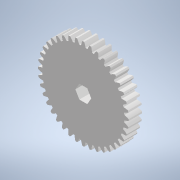
# Autodesk Inventor part: engranaje40
Saved by Autodesk Inventor 2022 (Build 260153000, 153)
## iProperties
Created: 2022-03-10
Part Number: engranaje40
Material: Generic
Document SubType Name: Modeling
Designer: katha
Density: 1 g/cm^3
Appearance: Default
Author: katha
Autodesk Inventor part; units mm, degrees
(part 1 of 4)
ref_plane "YZ Plane" through (0, 0, 0) normal (1, 0, 0) x (0, 1, 0)
ref_plane "XZ Plane" through (0, 0, 0) normal (0, 1, 0) x (-1, 0, 0)
ref_plane "XY Plane" through (0, 0, 0) normal (0, 0, 1) x (1, 0, 0)
sketch "Sketch4" plane through (0, 0, 0) normal (0, 0, 1) x (1, 0, 0)
  circle A0 centre (0, 0) radius 2
  circle A1 centre (0, 0) radius 2
  line L0 (20.6501, 2.8098) -> (20.4934, 2.709)
  line L1 (20.4934, 2.709) -> (20.3445, 2.6176)
  line L2 (20.3445, 2.6176) -> (20.199, 2.5324)
  line L3 (20.199, 2.5324) -> (20.06, 2.4548)
  line L4 (20.06, 2.4548) -> (19.7984, 2.3194)
  line L5 (19.7984, 2.3194) -> (19.561, 2.2088)
  line L6 (19.561, 2.2088) -> (19.3491, 2.1207)
  line L7 (19.3491, 2.1207) -> (19.1647, 2.0529)
  line L8 (19.1647, 2.0529) -> (19.0089, 2.0007)
  line L9 (19.0089, 2.0007) -> (18.9606, 1.9795)
  line L10 (18.9606, 1.9795) -> (18.9216, 1.9573)
  line L11 (18.9216, 1.9573) -> (18.8918, 1.9346)
  line L12 (18.8918, 1.9346) -> (18.8713, 1.9116)
  line L13 (18.8713, 1.9116) -> (18.86, 1.8888)
  line L14 (18.86, 1.8888) -> (18.8579, 1.8665)
  line L15 (18.8579, 1.8665) -> (18.8612, 1.833)
  line L16 (18.8612, 1.833) -> (18.8916, 1.4868)
  line L17 (18.8916, 1.4868) -> (18.9157, 1.1401)
  line L18 (18.9157, 1.1401) -> (18.9177, 1.1065)
  line L19 (18.9177, 1.1065) -> (18.9232, 1.0848)
  line L20 (18.9232, 1.0848) -> (18.938, 1.0641)
  line L21 (18.938, 1.0641) -> (18.9618, 1.0446)
  line L22 (18.9618, 1.0446) -> (18.9948, 1.0268)
  line L23 (18.9948, 1.0268) -> (19.0368, 1.011)
  line L24 (19.0368, 1.011) -> (19.0878, 0.9976)
  line L25 (19.0878, 0.9976) -> (19.2499, 0.9703)
  line L26 (19.2499, 0.9703) -> (19.4426, 0.9323)
  line L27 (19.4426, 0.9323) -> (19.6657, 0.8784)
  line L28 (19.6657, 0.8784) -> (19.9175, 0.8063)
  line L29 (19.9175, 0.8063) -> (20.1971, 0.7134)
  line L30 (20.1971, 0.7134) -> (20.3465, 0.6586)
  line L31 (20.3465, 0.6586) -> (20.5035, 0.5972)
  line L32 (20.5035, 0.5972) -> (20.6649, 0.5302)
  line L33 (20.6649, 0.5302) -> (20.8354, 0.4552)
  line L34 (20.8354, 0.4552) -> (20.9966, 0.3803)
  arc A2 (20.9966, -0.3803) -> (20.9966, 0.3803) centre (0, 0) ccw
  line L35 (20.9966, -0.3803) -> (20.8354, -0.4552)
  line L36 (20.8354, -0.4552) -> (20.6649, -0.5302)
  line L37 (20.6649, -0.5302) -> (20.5035, -0.5972)
  line L38 (20.5035, -0.5972) -> (20.3465, -0.6586)
  line L39 (20.3465, -0.6586) -> (20.1971, -0.7135)
  line L40 (20.1971, -0.7135) -> (19.9175, -0.8063)
  line L41 (19.9175, -0.8063) -> (19.6657, -0.8784)
  line L42 (19.6657, -0.8784) -> (19.4426, -0.9323)
  line L43 (19.4426, -0.9323) -> (19.2499, -0.9703)
  line L44 (19.2499, -0.9703) -> (19.0878, -0.9976)
  line L45 (19.0878, -0.9976) -> (19.0368, -1.011)
  line L46 (19.0368, -1.011) -> (18.9948, -1.0268)
  line L47 (18.9948, -1.0268) -> (18.9618, -1.0446)
  line L48 (18.9618, -1.0446) -> (18.938, -1.0641)
  line L49 (18.938, -1.0641) -> (18.9232, -1.0848)
  line L50 (18.9232, -1.0848) -> (18.9177, -1.1065)
  line L51 (18.9177, -1.1065) -> (18.9157, -1.1401)
  line L52 (18.9157, -1.1401) -> (18.8916, -1.4868)
  line L53 (18.8916, -1.4868) -> (18.8612, -1.833)
  line L54 (18.8612, -1.833) -> (18.8579, -1.8665)
  line L55 (18.8579, -1.8665) -> (18.86, -1.8888)
  line L56 (18.86, -1.8888) -> (18.8713, -1.9116)
  line L57 (18.8713, -1.9116) -> (18.8918, -1.9346)
  line L58 (18.8918, -1.9346) -> (18.9216, -1.9573)
  line L59 (18.9216, -1.9573) -> (18.9606, -1.9795)
  line L60 (18.9606, -1.9795) -> (19.0089, -2.0007)
  line L61 (19.0089, -2.0007) -> (19.1647, -2.053)
  line L62 (19.1647, -2.053) -> (19.3491, -2.1207)
  line L63 (19.3491, -2.1207) -> (19.561, -2.2088)
  line L64 (19.561, -2.2088) -> (19.7984, -2.3194)
  line L65 (19.7984, -2.3194) -> (20.06, -2.4548)
  line L66 (20.06, -2.4548) -> (20.199, -2.5324)
  line L67 (20.199, -2.5324) -> (20.3445, -2.6176)
  line L68 (20.3445, -2.6176) -> (20.4934, -2.709)
  line L69 (20.4934, -2.709) -> (20.6501, -2.8098)
  line L70 (20.6501, -2.8098) -> (20.7975, -2.909)
  arc A3 (20.6786, -3.6602) -> (20.7975, -2.909) centre (0, 0) ccw
  line L71 (20.6786, -3.6602) -> (20.5077, -3.709)
  line L72 (20.5077, -3.709) -> (20.3275, -3.7564)
  line L73 (20.3275, -3.7564) -> (20.1577, -3.7973)
  line L74 (20.1577, -3.7973) -> (19.993, -3.8334)
  line L75 (19.993, -3.8334) -> (19.8368, -3.8642)
  line L76 (19.8368, -3.8642) -> (19.5462, -3.9122)
  line L77 (19.5462, -3.9122) -> (19.2862, -3.944)
  line L78 (19.2862, -3.944) -> (19.0574, -3.9623)
  line L79 (19.0574, -3.9623) -> (18.8611, -3.9697)
  line L80 (18.8611, -3.9697) -> (18.6968, -3.9713)
  line L81 (18.6968, -3.9713) -> (18.6443, -3.9765)
  line L82 (18.6443, -3.9765) -> (18.6003, -3.9856)
  line L83 (18.6003, -3.9856) -> (18.565, -3.998)
  line L84 (18.565, -3.998) -> (18.5383, -4.0135)
  line L85 (18.5383, -4.0135) -> (18.5205, -4.0317)
  line L86 (18.5205, -4.0317) -> (18.5117, -4.0522)
  line L87 (18.5117, -4.0522) -> (18.5045, -4.0852)
  line L88 (18.5045, -4.0852) -> (18.4264, -4.4238)
  line L89 (18.4264, -4.4238) -> (18.3423, -4.761)
  line L90 (18.3423, -4.761) -> (18.3337, -4.7936)
  line L91 (18.3337, -4.7936) -> (18.3323, -4.8159)
  line L92 (18.3323, -4.8159) -> (18.3399, -4.8402)
  line L93 (18.3399, -4.8402) -> (18.3566, -4.8661)
  line L94 (18.3566, -4.8661) -> (18.3824, -4.8932)
  line L95 (18.3824, -4.8932) -> (18.4175, -4.9212)
  line L96 (18.4175, -4.9212) -> (18.4619, -4.9497)
  line L97 (18.4619, -4.9497) -> (18.6076, -5.0257)
  line L98 (18.6076, -5.0257) -> (18.7791, -5.1215)
  line L99 (18.7791, -5.1215) -> (18.9746, -5.2416)
  line L100 (18.9746, -5.2416) -> (19.1918, -5.388)
  line L101 (19.1918, -5.388) -> (19.429, -5.5627)
  line L102 (19.429, -5.5627) -> (19.5542, -5.661)
  line L103 (19.5542, -5.661) -> (19.6846, -5.768)
  line L104 (19.6846, -5.768) -> (19.8173, -5.8815)
  line L105 (19.8173, -5.8815) -> (19.9563, -6.0056)
  line L106 (19.9563, -6.0056) -> (20.0864, -6.1266)
  arc A4 (19.8514, -6.85) -> (20.0864, -6.1266) centre (0, 0) ccw
  line L107 (19.8514, -6.85) -> (19.675, -6.8714)
  line L108 (19.675, -6.8714) -> (19.4896, -6.8901)
  line L109 (19.4896, -6.8901) -> (19.3155, -6.9039)
  line L110 (19.3155, -6.9039) -> (19.1472, -6.9138)
  line L111 (19.1472, -6.9138) -> (18.9881, -6.9198)
  line L112 (18.9881, -6.9198) -> (18.6935, -6.9217)
  line L113 (18.6935, -6.9217) -> (18.4318, -6.9124)
  line L114 (18.4318, -6.9124) -> (18.203, -6.8948)
  line L115 (18.203, -6.8948) -> (18.0079, -6.8714)
  line L116 (18.0079, -6.8714) -> (17.8454, -6.8472)
  line L117 (17.8454, -6.8472) -> (17.7927, -6.8442)
  line L118 (17.7927, -6.8442) -> (17.7479, -6.8462)
  line L119 (17.7479, -6.8462) -> (17.711, -6.853)
  line L120 (17.711, -6.853) -> (17.6823, -6.8641)
  line L121 (17.6823, -6.8641) -> (17.6618, -6.8793)
  line L122 (17.6618, -6.8793) -> (17.6499, -6.8982)
  line L123 (17.6499, -6.8982) -> (17.6376, -6.9296)
  line L124 (17.6376, -6.9296) -> (17.5075, -7.2519)
  line L125 (17.5075, -7.2519) -> (17.3717, -7.5717)
  line L126 (17.3717, -7.5717) -> (17.3581, -7.6026)
  line L127 (17.3581, -7.6026) -> (17.3532, -7.6244)
  line L128 (17.3532, -7.6244) -> (17.3569, -7.6496)
  line L129 (17.3569, -7.6496) -> (17.3694, -7.6778)
  line L130 (17.3694, -7.6778) -> (17.3907, -7.7086)
  line L131 (17.3907, -7.7086) -> (17.4209, -7.7418)
  line L132 (17.4209, -7.7418) -> (17.4603, -7.7769)
  line L133 (17.4603, -7.7769) -> (17.5923, -7.8747)
  line L134 (17.5923, -7.8747) -> (17.7468, -7.9961)
  line L135 (17.7468, -7.9961) -> (17.9211, -8.1454)
  line L136 (17.9211, -8.1454) -> (18.1127, -8.324)
  line L137 (18.1127, -8.324) -> (18.3196, -8.5336)
  line L138 (18.3196, -8.5336) -> (18.4279, -8.6503)
  line L139 (18.4279, -8.6503) -> (18.5399, -8.7763)
  line L140 (18.5399, -8.7763) -> (18.6532, -8.9092)
  line L141 (18.6532, -8.9092) -> (18.7712, -9.0535)
  line L142 (18.7712, -9.0535) -> (18.8807, -9.1934)
  arc A5 (18.5354, -9.8711) -> (18.8807, -9.1934) centre (0, 0) ccw
  line L143 (18.5354, -9.8711) -> (18.3579, -9.8647)
  line L144 (18.3579, -9.8647) -> (18.1718, -9.8541)
  line L145 (18.1718, -9.8541) -> (17.9976, -9.8405)
  line L146 (17.9976, -9.8405) -> (17.8299, -9.8239)
  line L147 (17.8299, -9.8239) -> (17.6718, -9.805)
  line L148 (17.6718, -9.805) -> (17.3806, -9.7608)
  line L149 (17.3806, -9.7608) -> (17.1235, -9.7107)
  line L150 (17.1235, -9.7107) -> (16.9003, -9.6574)
  line L151 (16.9003, -9.6574) -> (16.7112, -9.6038)
  line L152 (16.7112, -9.6038) -> (16.5545, -9.5545)
  line L153 (16.5545, -9.5545) -> (16.503, -9.5433)
  line L154 (16.503, -9.5433) -> (16.4584, -9.5383)
  line L155 (16.4584, -9.5383) -> (16.4209, -9.5392)
  line L156 (16.4209, -9.5392) -> (16.3908, -9.5457)
  line L157 (16.3908, -9.5457) -> (16.3682, -9.5575)
  line L158 (16.3682, -9.5575) -> (16.3535, -9.5743)
  line L159 (16.3535, -9.5743) -> (16.3364, -9.6034)
  line L160 (16.3364, -9.6034) -> (16.1575, -9.9014)
  line L161 (16.1575, -9.9014) -> (15.9733, -10.196)
  line L162 (15.9733, -10.196) -> (15.9551, -10.2244)
  line L163 (15.9551, -10.2244) -> (15.9468, -10.2452)
  line L164 (15.9468, -10.2452) -> (15.9466, -10.2706)
  line L165 (15.9466, -10.2706) -> (15.9544, -10.3004)
  line L166 (15.9544, -10.3004) -> (15.9707, -10.3342)
  line L167 (15.9707, -10.3342) -> (15.9954, -10.3717)
  line L168 (15.9954, -10.3717) -> (16.0287, -10.4125)
  line L169 (16.0287, -10.4125) -> (16.1438, -10.5298)
  line L170 (16.1438, -10.5298) -> (16.2774, -10.6739)
  line L171 (16.2774, -10.6739) -> (16.4262, -10.8486)
  line L172 (16.4262, -10.8486) -> (16.5875, -11.0549)
  line L173 (16.5875, -11.0549) -> (16.7591, -11.2943)
  line L174 (16.7591, -11.2943) -> (16.8478, -11.4266)
  line L175 (16.8478, -11.4266) -> (16.9387, -11.5685)
  line L176 (16.9387, -11.5685) -> (17.0299, -11.7175)
  line L177 (17.0299, -11.7175) -> (17.1238, -11.8785)
  line L178 (17.1238, -11.8785) -> (17.2101, -12.0338)
  arc A6 (16.7631, -12.6491) -> (17.2101, -12.0338) centre (0, 0) ccw
  line L179 (16.7631, -12.6491) -> (16.5887, -12.615)
  line L180 (16.5887, -12.615) -> (16.4066, -12.5755)
  line L181 (16.4066, -12.5755) -> (16.2367, -12.5348)
  line L182 (16.2367, -12.5348) -> (16.0735, -12.4922)
  line L183 (16.0735, -12.4922) -> (15.9204, -12.4487)
  line L184 (15.9204, -12.4487) -> (15.6397, -12.3595)
  line L185 (15.6397, -12.3595) -> (15.3936, -12.2699)
  line L186 (15.3936, -12.2699) -> (15.1815, -12.1823)
  line L187 (15.1815, -12.1823) -> (15.0031, -12.0998)
  line L188 (15.0031, -12.0998) -> (14.856, -12.0266)
  line L189 (14.856, -12.0266) -> (14.8069, -12.0075)
  line L190 (14.8069, -12.0075) -> (14.7636, -11.9956)
  line L191 (14.7636, -11.9956) -> (14.7265, -11.9906)
  line L192 (14.7265, -11.9906) -> (14.6957, -11.9923)
  line L193 (14.6957, -11.9923) -> (14.6716, -12.0004)
  line L194 (14.6716, -12.0004) -> (14.6544, -12.0147)
  line L195 (14.6544, -12.0147) -> (14.633, -12.0408)
  line L196 (14.633, -12.0408) -> (14.4097, -12.307)
  line L197 (14.4097, -12.307) -> (14.1816, -12.5693)
  line L198 (14.1816, -12.5693) -> (14.1592, -12.5944)
  line L199 (14.1592, -12.5944) -> (14.1478, -12.6137)
  line L200 (14.1478, -12.6137) -> (14.1436, -12.6388)
  line L201 (14.1436, -12.6388) -> (14.1467, -12.6694)
  line L202 (14.1467, -12.6694) -> (14.1574, -12.7053)
  line L203 (14.1574, -12.7053) -> (14.1759, -12.7462)
  line L204 (14.1759, -12.7462) -> (14.2025, -12.7918)
  line L205 (14.2025, -12.7918) -> (14.2978, -12.9256)
  line L206 (14.2978, -12.9256) -> (14.4072, -13.0888)
  line L207 (14.4072, -13.0888) -> (14.5269, -13.2846)
  line L208 (14.5269, -13.2846) -> (14.654, -13.5137)
  line L209 (14.654, -13.5137) -> (14.786, -13.777)
  line L210 (14.786, -13.777) -> (14.8529, -13.9214)
  line L211 (14.8529, -13.9214) -> (14.9205, -14.0759)
  line L212 (14.9205, -14.0759) -> (14.9872, -14.2373)
  line L213 (14.9872, -14.2373) -> (15.0547, -14.411)
  line L214 (15.0547, -14.411) -> (15.1157, -14.5779)
  arc A7 (14.5779, -15.1157) -> (15.1157, -14.5779) centre (0, 0) ccw
  line L215 (14.5779, -15.1157) -> (14.411, -15.0547)
  line L216 (14.411, -15.0547) -> (14.2373, -14.9872)
  line L217 (14.2373, -14.9872) -> (14.0759, -14.9205)
  line L218 (14.0759, -14.9205) -> (13.9214, -14.8529)
  line L219 (13.9214, -14.8529) -> (13.777, -14.786)
  line L220 (13.777, -14.786) -> (13.5137, -14.654)
  line L221 (13.5137, -14.654) -> (13.2846, -14.5269)
  line L222 (13.2846, -14.5269) -> (13.0888, -14.4072)
  line L223 (13.0888, -14.4072) -> (12.9256, -14.2978)
  line L224 (12.9256, -14.2978) -> (12.7918, -14.2025)
  line L225 (12.7918, -14.2025) -> (12.7462, -14.176)
  line L226 (12.7462, -14.176) -> (12.7053, -14.1574)
  line L227 (12.7053, -14.1574) -> (12.6694, -14.1467)
  line L228 (12.6694, -14.1467) -> (12.6388, -14.1436)
  line L229 (12.6388, -14.1436) -> (12.6137, -14.1478)
  line L230 (12.6137, -14.1478) -> (12.5944, -14.1592)
  line L231 (12.5944, -14.1592) -> (12.5693, -14.1816)
  line L232 (12.5693, -14.1816) -> (12.307, -14.4097)
  line L233 (12.307, -14.4097) -> (12.0408, -14.633)
  line L234 (12.0408, -14.633) -> (12.0147, -14.6544)
  line L235 (12.0147, -14.6544) -> (12.0004, -14.6716)
  line L236 (12.0004, -14.6716) -> (11.9923, -14.6957)
  line L237 (11.9923, -14.6957) -> (11.9906, -14.7265)
  line L238 (11.9906, -14.7265) -> (11.9956, -14.7636)
  line L239 (11.9956, -14.7636) -> (12.0075, -14.8069)
  line L240 (12.0075, -14.8069) -> (12.0266, -14.856)
  line L241 (12.0266, -14.856) -> (12.0998, -15.0031)
  line L242 (12.0998, -15.0031) -> (12.1823, -15.1815)
  line L243 (12.1823, -15.1815) -> (12.2698, -15.3936)
  line L244 (12.2698, -15.3936) -> (12.3595, -15.6397)
  line L245 (12.3595, -15.6397) -> (12.4487, -15.9204)
  line L246 (12.4487, -15.9204) -> (12.4922, -16.0736)
  line L247 (12.4922, -16.0736) -> (12.5348, -16.2367)
  line L248 (12.5348, -16.2367) -> (12.5755, -16.4066)
  line L249 (12.5755, -16.4066) -> (12.615, -16.5887)
  line L250 (12.615, -16.5887) -> (12.6491, -16.7631)
  arc A8 (12.0338, -17.2101) -> (12.6491, -16.7631) centre (0, 0) ccw
  line L251 (12.0338, -17.2101) -> (11.8785, -17.1238)
  line L252 (11.8785, -17.1238) -> (11.7175, -17.0299)
  line L253 (11.7175, -17.0299) -> (11.5685, -16.9387)
  line L254 (11.5685, -16.9387) -> (11.4265, -16.8478)
  line L255 (11.4265, -16.8478) -> (11.2943, -16.7591)
  line L256 (11.2943, -16.7591) -> (11.0549, -16.5875)
  line L257 (11.0549, -16.5875) -> (10.8486, -16.4262)
  line L258 (10.8486, -16.4262) -> (10.6739, -16.2774)
  line L259 (10.6739, -16.2774) -> (10.5298, -16.1438)
  line L260 (10.5298, -16.1438) -> (10.4125, -16.0287)
  line L261 (10.4125, -16.0287) -> (10.3717, -15.9954)
  line L262 (10.3717, -15.9954) -> (10.3342, -15.9707)
  line L263 (10.3342, -15.9707) -> (10.3004, -15.9544)
  line L264 (10.3004, -15.9544) -> (10.2706, -15.9466)
  line L265 (10.2706, -15.9466) -> (10.2452, -15.9469)
  line L266 (10.2452, -15.9469) -> (10.2244, -15.9551)
  line L267 (10.2244, -15.9551) -> (10.196, -15.9733)
  line L268 (10.196, -15.9733) -> (9.9014, -16.1575)
  line L269 (9.9014, -16.1575) -> (9.6034, -16.3365)
  line L270 (9.6034, -16.3365) -> (9.5743, -16.3535)
  line L271 (9.5743, -16.3535) -> (9.5575, -16.3682)
  line L272 (9.5575, -16.3682) -> (9.5457, -16.3908)
  line L273 (9.5457, -16.3908) -> (9.5392, -16.4209)
  line L274 (9.5392, -16.4209) -> (9.5383, -16.4584)
  line L275 (9.5383, -16.4584) -> (9.5433, -16.503)
  line L276 (9.5433, -16.503) -> (9.5545, -16.5545)
  line L277 (9.5545, -16.5545) -> (9.6038, -16.7112)
  line L278 (9.6038, -16.7112) -> (9.6574, -16.9003)
  line L279 (9.6574, -16.9003) -> (9.7107, -17.1235)
  line L280 (9.7107, -17.1235) -> (9.7608, -17.3806)
  line L281 (9.7608, -17.3806) -> (9.805, -17.6718)
  line L282 (9.805, -17.6718) -> (9.8239, -17.8299)
  line L283 (9.8239, -17.8299) -> (9.8405, -17.9977)
  line L284 (9.8405, -17.9977) -> (9.8541, -18.1718)
  line L285 (9.8541, -18.1718) -> (9.8647, -18.3579)
  line L286 (9.8647, -18.3579) -> (9.8711, -18.5354)
  arc A9 (9.1934, -18.8807) -> (9.8711, -18.5354) centre (0, 0) ccw
  line L287 (9.1934, -18.8807) -> (9.0535, -18.7712)
  line L288 (9.0535, -18.7712) -> (8.9092, -18.6532)
  line L289 (8.9092, -18.6532) -> (8.7763, -18.5399)
  line L290 (8.7763, -18.5399) -> (8.6503, -18.4279)
  line L291 (8.6503, -18.4279) -> (8.5336, -18.3196)
  line L292 (8.5336, -18.3196) -> (8.324, -18.1127)
  line L293 (8.324, -18.1127) -> (8.1454, -17.9211)
  line L294 (8.1454, -17.9211) -> (7.9961, -17.7468)
  line L295 (7.9961, -17.7468) -> (7.8747, -17.5923)
  line L296 (7.8747, -17.5923) -> (7.7769, -17.4603)
  line L297 (7.7769, -17.4603) -> (7.7418, -17.4209)
  line L298 (7.7418, -17.4209) -> (7.7086, -17.3907)
  line L299 (7.7086, -17.3907) -> (7.6778, -17.3694)
  line L300 (7.6778, -17.3694) -> (7.6496, -17.3569)
  line L301 (7.6496, -17.3569) -> (7.6244, -17.3532)
  line L302 (7.6244, -17.3532) -> (7.6026, -17.3581)
  line L303 (7.6026, -17.3581) -> (7.5717, -17.3717)
  line L304 (7.5717, -17.3717) -> (7.2519, -17.5075)
  line L305 (7.2519, -17.5075) -> (6.9296, -17.6376)
  line L306 (6.9296, -17.6376) -> (6.8982, -17.6499)
  line L307 (6.8982, -17.6499) -> (6.8793, -17.6618)
  line L308 (6.8793, -17.6618) -> (6.8641, -17.6823)
  line L309 (6.8641, -17.6823) -> (6.853, -17.711)
  line L310 (6.853, -17.711) -> (6.8462, -17.7479)
  line L311 (6.8462, -17.7479) -> (6.8442, -17.7927)
  line L312 (6.8442, -17.7927) -> (6.8472, -17.8454)
  line L313 (6.8472, -17.8454) -> (6.8714, -18.0079)
  line L314 (6.8714, -18.0079) -> (6.8947, -18.203)
  line L315 (6.8947, -18.203) -> (6.9124, -18.4318)
  line L316 (6.9124, -18.4318) -> (6.9217, -18.6935)
  line L317 (6.9217, -18.6935) -> (6.9198, -18.9881)
  line L318 (6.9198, -18.9881) -> (6.9138, -19.1472)
  line L319 (6.9138, -19.1472) -> (6.9039, -19.3155)
  line L320 (6.9039, -19.3155) -> (6.8901, -19.4896)
  line L321 (6.8901, -19.4896) -> (6.8714, -19.675)
  line L322 (6.8714, -19.675) -> (6.85, -19.8514)
  arc A10 (6.1266, -20.0864) -> (6.85, -19.8514) centre (0, 0) ccw
  line L323 (6.1266, -20.0864) -> (6.0056, -19.9563)
  line L324 (6.0056, -19.9563) -> (5.8815, -19.8173)
  line L325 (5.8815, -19.8173) -> (5.768, -19.6846)
  line L326 (5.768, -19.6846) -> (5.661, -19.5542)
  line L327 (5.661, -19.5542) -> (5.5627, -19.429)
  line L328 (5.5627, -19.429) -> (5.388, -19.1919)
  line L329 (5.388, -19.1919) -> (5.2416, -18.9746)
  line L330 (5.2416, -18.9746) -> (5.1215, -18.7791)
  line L331 (5.1215, -18.7791) -> (5.0257, -18.6076)
  line L332 (5.0257, -18.6076) -> (4.9497, -18.4619)
  line L333 (4.9497, -18.4619) -> (4.9212, -18.4175)
  line L334 (4.9212, -18.4175) -> (4.8932, -18.3825)
  line L335 (4.8932, -18.3825) -> (4.8661, -18.3566)
  line L336 (4.8661, -18.3566) -> (4.8402, -18.3399)
  line L337 (4.8402, -18.3399) -> (4.8159, -18.3323)
  line L338 (4.8159, -18.3323) -> (4.7936, -18.3337)
  line L339 (4.7936, -18.3337) -> (4.761, -18.3423)
  line L340 (4.761, -18.3423) -> (4.4238, -18.4264)
  line L341 (4.4238, -18.4264) -> (4.0852, -18.5045)
  line L342 (4.0852, -18.5045) -> (4.0522, -18.5117)
  line L343 (4.0522, -18.5117) -> (4.0317, -18.5206)
  line L344 (4.0317, -18.5206) -> (4.0135, -18.5383)
  line L345 (4.0135, -18.5383) -> (3.998, -18.565)
  line L346 (3.998, -18.565) -> (3.9856, -18.6004)
  line L347 (3.9856, -18.6004) -> (3.9765, -18.6443)
  line L348 (3.9765, -18.6443) -> (3.9713, -18.6968)
  line L349 (3.9713, -18.6968) -> (3.9697, -18.8611)
  line L350 (3.9697, -18.8611) -> (3.9623, -19.0574)
  line L351 (3.9623, -19.0574) -> (3.944, -19.2862)
  line L352 (3.944, -19.2862) -> (3.9122, -19.5462)
  line L353 (3.9122, -19.5462) -> (3.8642, -19.8368)
  line L354 (3.8642, -19.8368) -> (3.8334, -19.993)
  line L355 (3.8334, -19.993) -> (3.7973, -20.1577)
  line L356 (3.7973, -20.1577) -> (3.7564, -20.3275)
  line L357 (3.7564, -20.3275) -> (3.709, -20.5077)
  line L358 (3.709, -20.5077) -> (3.6602, -20.6786)
  arc A11 (2.909, -20.7975) -> (3.6602, -20.6786) centre (0, 0) ccw
  line L359 (2.909, -20.7975) -> (2.8098, -20.6501)
  line L360 (2.8098, -20.6501) -> (2.709, -20.4934)
  line L361 (2.709, -20.4934) -> (2.6176, -20.3445)
  line L362 (2.6176, -20.3445) -> (2.5324, -20.199)
  line L363 (2.5324, -20.199) -> (2.4548, -20.06)
  line L364 (2.4548, -20.06) -> (2.3194, -19.7984)
  line L365 (2.3194, -19.7984) -> (2.2088, -19.561)
  line L366 (2.2088, -19.561) -> (2.1207, -19.3491)
  line L367 (2.1207, -19.3491) -> (2.0529, -19.1647)
  line L368 (2.0529, -19.1647) -> (2.0007, -19.0089)
  line L369 (2.0007, -19.0089) -> (1.9795, -18.9606)
  line L370 (1.9795, -18.9606) -> (1.9573, -18.9216)
  line L371 (1.9573, -18.9216) -> (1.9346, -18.8918)
  line L372 (1.9346, -18.8918) -> (1.9116, -18.8713)
  line L373 (1.9116, -18.8713) -> (1.8888, -18.86)
  line L374 (1.8888, -18.86) -> (1.8665, -18.8579)
  line L375 (1.8665, -18.8579) -> (1.833, -18.8612)
  line L376 (1.833, -18.8612) -> (1.4868, -18.8916)
  line L377 (1.4868, -18.8916) -> (1.1401, -18.9157)
  line L378 (1.1401, -18.9157) -> (1.1065, -18.9177)
  line L379 (1.1065, -18.9177) -> (1.0848, -18.9232)
  line L380 (1.0848, -18.9232) -> (1.0641, -18.938)
  line L381 (1.0641, -18.938) -> (1.0446, -18.9618)
  line L382 (1.0446, -18.9618) -> (1.0268, -18.9948)
  line L383 (1.0268, -18.9948) -> (1.011, -19.0369)
  line L384 (1.011, -19.0369) -> (0.9976, -19.0878)
  line L385 (0.9976, -19.0878) -> (0.9703, -19.2499)
  line L386 (0.9703, -19.2499) -> (0.9323, -19.4427)
  line L387 (0.9323, -19.4427) -> (0.8784, -19.6657)
  line L388 (0.8784, -19.6657) -> (0.8063, -19.9175)
  line L389 (0.8063, -19.9175) -> (0.7135, -20.1971)
  line L390 (0.7135, -20.1971) -> (0.6586, -20.3465)
  line L391 (0.6586, -20.3465) -> (0.5972, -20.5035)
  line L392 (0.5972, -20.5035) -> (0.5302, -20.6649)
  line L393 (0.5302, -20.6649) -> (0.4552, -20.8354)
  line L394 (0.4552, -20.8354) -> (0.3803, -20.9966)
  arc A12 (-0.3803, -20.9966) -> (0.3803, -20.9966) centre (0, 0) ccw
  line L395 (-0.3803, -20.9966) -> (-0.4552, -20.8354)
  line L396 (-0.4552, -20.8354) -> (-0.5302, -20.6649)
  line L397 (-0.5302, -20.6649) -> (-0.5972, -20.5035)
  line L398 (-0.5972, -20.5035) -> (-0.6586, -20.3465)
  line L399 (-0.6586, -20.3465) -> (-0.7135, -20.1971)
  line L400 (-0.7135, -20.1971) -> (-0.8063, -19.9175)
  line L401 (-0.8063, -19.9175) -> (-0.8784, -19.6657)
  line L402 (-0.8784, -19.6657) -> (-0.9323, -19.4426)
  line L403 (-0.9323, -19.4426) -> (-0.9703, -19.2499)
  line L404 (-0.9703, -19.2499) -> (-0.9976, -19.0878)
  line L405 (-0.9976, -19.0878) -> (-1.011, -19.0369)
  line L406 (-1.011, -19.0369) -> (-1.0268, -18.9948)
  line L407 (-1.0268, -18.9948) -> (-1.0446, -18.9618)
  line L408 (-1.0446, -18.9618) -> (-1.0641, -18.938)
  line L409 (-1.0641, -18.938) -> (-1.0848, -18.9232)
  line L410 (-1.0848, -18.9232) -> (-1.1065, -18.9177)
  line L411 (-1.1065, -18.9177) -> (-1.1401, -18.9157)
  line L412 (-1.1401, -18.9157) -> (-1.4868, -18.8916)
  line L413 (-1.4868, -18.8916) -> (-1.833, -18.8612)
  line L414 (-1.833, -18.8612) -> (-1.8665, -18.8579)
  line L415 (-1.8665, -18.8579) -> (-1.8888, -18.86)
  line L416 (-1.8888, -18.86) -> (-1.9116, -18.8713)
  line L417 (-1.9116, -18.8713) -> (-1.9346, -18.8918)
  line L418 (-1.9346, -18.8918) -> (-1.9573, -18.9216)
  line L419 (-1.9573, -18.9216) -> (-1.9795, -18.9606)
  line L420 (-1.9795, -18.9606) -> (-2.0007, -19.0089)
  line L421 (-2.0007, -19.0089) -> (-2.0529, -19.1647)
  line L422 (-2.0529, -19.1647) -> (-2.1207, -19.3491)
  line L423 (-2.1207, -19.3491) -> (-2.2088, -19.561)
  line L424 (-2.2088, -19.561) -> (-2.3194, -19.7984)
  line L425 (-2.3194, -19.7984) -> (-2.4548, -20.06)
  line L426 (-2.4548, -20.06) -> (-2.5324, -20.199)
  line L427 (-2.5324, -20.199) -> (-2.6176, -20.3445)
  line L428 (-2.6176, -20.3445) -> (-2.709, -20.4934)
  line L429 (-2.709, -20.4934) -> (-2.8098, -20.6501)
  line L430 (-2.8098, -20.6501) -> (-2.909, -20.7975)
  arc A13 (-3.6602, -20.6786) -> (-2.909, -20.7975) centre (0, 0) ccw
  line L431 (-3.6602, -20.6786) -> (-3.7089, -20.5077)
  line L432 (-3.7089, -20.5077) -> (-3.7564, -20.3275)
  line L433 (-3.7564, -20.3275) -> (-3.7973, -20.1577)
  line L434 (-3.7973, -20.1577) -> (-3.8334, -19.993)
  line L435 (-3.8334, -19.993) -> (-3.8642, -19.8368)
  line L436 (-3.8642, -19.8368) -> (-3.9122, -19.5462)
  line L437 (-3.9122, -19.5462) -> (-3.944, -19.2862)
  line L438 (-3.944, -19.2862) -> (-3.9623, -19.0574)
  line L439 (-3.9623, -19.0574) -> (-3.9697, -18.8611)
  line L440 (-3.9697, -18.8611) -> (-3.9713, -18.6968)
  line L441 (-3.9713, -18.6968) -> (-3.9765, -18.6443)
  line L442 (-3.9765, -18.6443) -> (-3.9856, -18.6004)
  line L443 (-3.9856, -18.6004) -> (-3.998, -18.565)
  line L444 (-3.998, -18.565) -> (-4.0135, -18.5383)
  line L445 (-4.0135, -18.5383) -> (-4.0317, -18.5206)
  line L446 (-4.0317, -18.5206) -> (-4.0522, -18.5117)
  line L447 (-4.0522, -18.5117) -> (-4.0852, -18.5045)
  line L448 (-4.0852, -18.5045) -> (-4.4238, -18.4264)
  line L449 (-4.4238, -18.4264) -> (-4.761, -18.3423)
  line L450 (-4.761, -18.3423) -> (-4.7936, -18.3337)
  line L451 (-4.7936, -18.3337) -> (-4.8159, -18.3323)
  line L452 (-4.8159, -18.3323) -> (-4.8402, -18.3399)
  line L453 (-4.8402, -18.3399) -> (-4.8661, -18.3566)
  line L454 (-4.8661, -18.3566) -> (-4.8932, -18.3825)
  line L455 (-4.8932, -18.3825) -> (-4.9212, -18.4175)
  line L456 (-4.9212, -18.4175) -> (-4.9497, -18.4619)
  line L457 (-4.9497, -18.4619) -> (-5.0257, -18.6076)
  line L458 (-5.0257, -18.6076) -> (-5.1215, -18.7791)
  line L459 (-5.1215, -18.7791) -> (-5.2416, -18.9746)
  line L460 (-5.2416, -18.9746) -> (-5.388, -19.1919)
  line L461 (-5.388, -19.1919) -> (-5.5627, -19.429)
  line L462 (-5.5627, -19.429) -> (-5.661, -19.5542)
  line L463 (-5.661, -19.5542) -> (-5.7679, -19.6846)
  line L464 (-5.7679, -19.6846) -> (-5.8815, -19.8173)
  line L465 (-5.8815, -19.8173) -> (-6.0056, -19.9563)
  line L466 (-6.0056, -19.9563) -> (-6.1266, -20.0864)
  arc A14 (-6.85, -19.8514) -> (-6.1266, -20.0864) centre (0, 0) ccw
  line L467 (-6.85, -19.8514) -> (-6.8714, -19.675)
  line L468 (-6.8714, -19.675) -> (-6.8901, -19.4896)
  line L469 (-6.8901, -19.4896) -> (-6.9039, -19.3155)
  line L470 (-6.9039, -19.3155) -> (-6.9138, -19.1472)
  line L471 (-6.9138, -19.1472) -> (-6.9198, -18.9881)
  line L472 (-6.9198, -18.9881) -> (-6.9217, -18.6935)
  line L473 (-6.9217, -18.6935) -> (-6.9124, -18.4318)
  line L474 (-6.9124, -18.4318) -> (-6.8947, -18.203)
  line L475 (-6.8947, -18.203) -> (-6.8714, -18.0079)
  line L476 (-6.8714, -18.0079) -> (-6.8472, -17.8454)
  line L477 (-6.8472, -17.8454) -> (-6.8442, -17.7927)
  line L478 (-6.8442, -17.7927) -> (-6.8462, -17.7479)
  line L479 (-6.8462, -17.7479) -> (-6.853, -17.711)
  line L480 (-6.853, -17.711) -> (-6.8641, -17.6823)
  line L481 (-6.8641, -17.6823) -> (-6.8793, -17.6618)
  line L482 (-6.8793, -17.6618) -> (-6.8982, -17.6499)
  line L483 (-6.8982, -17.6499) -> (-6.9296, -17.6376)
  line L484 (-6.9296, -17.6376) -> (-7.2519, -17.5075)
  line L485 (-7.2519, -17.5075) -> (-7.5717, -17.3717)
  line L486 (-7.5717, -17.3717) -> (-7.6026, -17.3581)
  line L487 (-7.6026, -17.3581) -> (-7.6244, -17.3532)
  line L488 (-7.6244, -17.3532) -> (-7.6496, -17.3569)
  line L489 (-7.6496, -17.3569) -> (-7.6778, -17.3694)
  line L490 (-7.6778, -17.3694) -> (-7.7086, -17.3907)
  line L491 (-7.7086, -17.3907) -> (-7.7418, -17.4209)
  line L492 (-7.7418, -17.4209) -> (-7.7769, -17.4603)
  line L493 (-7.7769, -17.4603) -> (-7.8747, -17.5923)
  line L494 (-7.8747, -17.5923) -> (-7.9961, -17.7468)
  line L495 (-7.9961, -17.7468) -> (-8.1454, -17.9211)
  line L496 (-8.1454, -17.9211) -> (-8.3239, -18.1127)
  line L497 (-8.3239, -18.1127) -> (-8.5336, -18.3196)
  line L498 (-8.5336, -18.3196) -> (-8.6503, -18.4279)
  line L499 (-8.6503, -18.4279) -> (-8.7763, -18.5399)
  line L500 (-8.7763, -18.5399) -> (-8.9092, -18.6532)
  line L501 (-8.9092, -18.6532) -> (-9.0535, -18.7712)
  line L502 (-9.0535, -18.7712) -> (-9.1934, -18.8807)
  arc A15 (-9.8711, -18.5354) -> (-9.1934, -18.8807) centre (0, 0) ccw
  line L503 (-9.8711, -18.5354) -> (-9.8647, -18.3579)
  line L504 (-9.8647, -18.3579) -> (-9.8541, -18.1718)
  line L505 (-9.8541, -18.1718) -> (-9.8405, -17.9977)
  line L506 (-9.8405, -17.9977) -> (-9.8239, -17.8299)
  line L507 (-9.8239, -17.8299) -> (-9.805, -17.6718)
  line L508 (-9.805, -17.6718) -> (-9.7608, -17.3806)
  line L509 (-9.7608, -17.3806) -> (-9.7107, -17.1235)
  line L510 (-9.7107, -17.1235) -> (-9.6574, -16.9003)
  line L511 (-9.6574, -16.9003) -> (-9.6038, -16.7112)
  line L512 (-9.6038, -16.7112) -> (-9.5545, -16.5545)
  line L513 (-9.5545, -16.5545) -> (-9.5433, -16.503)
  line L514 (-9.5433, -16.503) -> (-9.5383, -16.4584)
  line L515 (-9.5383, -16.4584) -> (-9.5392, -16.4209)
  line L516 (-9.5392, -16.4209) -> (-9.5457, -16.3908)
  line L517 (-9.5457, -16.3908) -> (-9.5575, -16.3682)
  line L518 (-9.5575, -16.3682) -> (-9.5743, -16.3535)
  line L519 (-9.5743, -16.3535) -> (-9.6034, -16.3365)
  line L520 (-9.6034, -16.3365) -> (-9.9013, -16.1575)
  line L521 (-9.9013, -16.1575) -> (-10.196, -15.9733)
  line L522 (-10.196, -15.9733) -> (-10.2244, -15.9551)
  line L523 (-10.2244, -15.9551) -> (-10.2452, -15.9469)
  line L524 (-10.2452, -15.9469) -> (-10.2706, -15.9466)
  line L525 (-10.2706, -15.9466) -> (-10.3004, -15.9544)
  line L526 (-10.3004, -15.9544) -> (-10.3342, -15.9707)
  line L527 (-10.3342, -15.9707) -> (-10.3717, -15.9954)
  line L528 (-10.3717, -15.9954) -> (-10.4125, -16.0287)
  line L529 (-10.4125, -16.0287) -> (-10.5298, -16.1438)
  line L530 (-10.5298, -16.1438) -> (-10.6739, -16.2774)
  line L531 (-10.6739, -16.2774) -> (-10.8486, -16.4262)
  line L532 (-10.8486, -16.4262) -> (-11.0549, -16.5875)
  line L533 (-11.0549, -16.5875) -> (-11.2943, -16.7591)
  line L534 (-11.2943, -16.7591) -> (-11.4265, -16.8478)
  line L535 (-11.4265, -16.8478) -> (-11.5685, -16.9387)
  line L536 (-11.5685, -16.9387) -> (-11.7175, -17.0299)
  line L537 (-11.7175, -17.0299) -> (-11.8785, -17.1238)
  line L538 (-11.8785, -17.1238) -> (-12.0338, -17.2101)
  arc A16 (-12.6491, -16.7631) -> (-12.0338, -17.2101) centre (0, 0) ccw
  line L539 (-12.6491, -16.7631) -> (-12.615, -16.5887)
  line L540 (-12.615, -16.5887) -> (-12.5755, -16.4066)
  line L541 (-12.5755, -16.4066) -> (-12.5348, -16.2367)
  line L542 (-12.5348, -16.2367) -> (-12.4922, -16.0736)
  line L543 (-12.4922, -16.0736) -> (-12.4487, -15.9204)
  line L544 (-12.4487, -15.9204) -> (-12.3595, -15.6397)
  line L545 (-12.3595, -15.6397) -> (-12.2698, -15.3936)
  line L546 (-12.2698, -15.3936) -> (-12.1823, -15.1815)
  line L547 (-12.1823, -15.1815) -> (-12.0998, -15.0031)
  line L548 (-12.0998, -15.0031) -> (-12.0266, -14.856)
  line L549 (-12.0266, -14.856) -> (-12.0075, -14.8069)
  line L550 (-12.0075, -14.8069) -> (-11.9956, -14.7636)
  line L551 (-11.9956, -14.7636) -> (-11.9906, -14.7265)
  line L552 (-11.9906, -14.7265) -> (-11.9923, -14.6957)
  line L553 (-11.9923, -14.6957) -> (-12.0004, -14.6716)
  line L554 (-12.0004, -14.6716) -> (-12.0147, -14.6544)
  line L555 (-12.0147, -14.6544) -> (-12.0408, -14.633)
  line L556 (-12.0408, -14.633) -> (-12.307, -14.4097)
  line L557 (-12.307, -14.4097) -> (-12.5693, -14.1816)
  line L558 (-12.5693, -14.1816) -> (-12.5944, -14.1592)
  line L559 (-12.5944, -14.1592) -> (-12.6137, -14.1478)
  line L560 (-12.6137, -14.1478) -> (-12.6387, -14.1436)
  line L561 (-12.6387, -14.1436) -> (-12.6694, -14.1467)
  line L562 (-12.6694, -14.1467) -> (-12.7053, -14.1574)
  line L563 (-12.7053, -14.1574) -> (-12.7462, -14.176)
  line L564 (-12.7462, -14.176) -> (-12.7918, -14.2025)
  line L565 (-12.7918, -14.2025) -> (-12.9256, -14.2978)
  line L566 (-12.9256, -14.2978) -> (-13.0888, -14.4072)
  line L567 (-13.0888, -14.4072) -> (-13.2846, -14.5269)
  line L568 (-13.2846, -14.5269) -> (-13.5137, -14.654)
  line L569 (-13.5137, -14.654) -> (-13.777, -14.786)
  line L570 (-13.777, -14.786) -> (-13.9214, -14.8529)
  line L571 (-13.9214, -14.8529) -> (-14.0759, -14.9205)
  line L572 (-14.0759, -14.9205) -> (-14.2373, -14.9872)
  line L573 (-14.2373, -14.9872) -> (-14.411, -15.0547)
  line L574 (-14.411, -15.0547) -> (-14.5779, -15.1157)
  arc A17 (-15.1157, -14.5779) -> (-14.5779, -15.1157) centre (0, 0) ccw
  line L575 (-15.1157, -14.5779) -> (-15.0547, -14.411)
  line L576 (-15.0547, -14.411) -> (-14.9872, -14.2373)
  line L577 (-14.9872, -14.2373) -> (-14.9205, -14.0759)
  line L578 (-14.9205, -14.0759) -> (-14.8529, -13.9214)
  line L579 (-14.8529, -13.9214) -> (-14.786, -13.777)
  line L580 (-14.786, -13.777) -> (-14.654, -13.5137)
  line L581 (-14.654, -13.5137) -> (-14.5269, -13.2846)
  line L582 (-14.5269, -13.2846) -> (-14.4072, -13.0888)
  line L583 (-14.4072, -13.0888) -> (-14.2978, -12.9256)
  line L584 (-14.2978, -12.9256) -> (-14.2025, -12.7918)
  line L585 (-14.2025, -12.7918) -> (-14.1759, -12.7462)
  line L586 (-14.1759, -12.7462) -> (-14.1574, -12.7053)
  line L587 (-14.1574, -12.7053) -> (-14.1467, -12.6694)
  line L588 (-14.1467, -12.6694) -> (-14.1436, -12.6388)
  line L589 (-14.1436, -12.6388) -> (-14.1478, -12.6137)
  line L590 (-14.1478, -12.6137) -> (-14.1592, -12.5944)
  line L591 (-14.1592, -12.5944) -> (-14.1816, -12.5693)
  line L592 (-14.1816, -12.5693) -> (-14.4097, -12.307)
  line L593 (-14.4097, -12.307) -> (-14.633, -12.0408)
  line L594 (-14.633, -12.0408) -> (-14.6544, -12.0147)
  line L595 (-14.6544, -12.0147) -> (-14.6716, -12.0004)
  line L596 (-14.6716, -12.0004) -> (-14.6957, -11.9923)
  line L597 (-14.6957, -11.9923) -> (-14.7265, -11.9906)
  line L598 (-14.7265, -11.9906) -> (-14.7636, -11.9956)
  line L599 (-14.7636, -11.9956) -> (-14.8069, -12.0075)
  line L600 (-14.8069, -12.0075) -> (-14.856, -12.0266)
  line L601 (-14.856, -12.0266) -> (-15.0031, -12.0998)
  line L602 (-15.0031, -12.0998) -> (-15.1815, -12.1823)
  line L603 (-15.1815, -12.1823) -> (-15.3936, -12.2699)
  line L604 (-15.3936, -12.2699) -> (-15.6397, -12.3595)
  line L605 (-15.6397, -12.3595) -> (-15.9204, -12.4487)
  line L606 (-15.9204, -12.4487) -> (-16.0735, -12.4922)
  line L607 (-16.0735, -12.4922) -> (-16.2367, -12.5348)
  line L608 (-16.2367, -12.5348) -> (-16.4066, -12.5755)
  line L609 (-16.4066, -12.5755) -> (-16.5887, -12.615)
  line L610 (-16.5887, -12.615) -> (-16.763, -12.6491)
  arc A18 (-17.2101, -12.0338) -> (-16.763, -12.6491) centre (0, 0) ccw
  line L611 (-17.2101, -12.0338) -> (-17.1238, -11.8785)
  line L612 (-17.1238, -11.8785) -> (-17.0299, -11.7175)
  line L613 (-17.0299, -11.7175) -> (-16.9387, -11.5685)
  line L614 (-16.9387, -11.5685) -> (-16.8478, -11.4266)
  line L615 (-16.8478, -11.4266) -> (-16.7591, -11.2943)
  line L616 (-16.7591, -11.2943) -> (-16.5875, -11.0549)
  line L617 (-16.5875, -11.0549) -> (-16.4262, -10.8486)
  line L618 (-16.4262, -10.8486) -> (-16.2774, -10.6739)
  line L619 (-16.2774, -10.6739) -> (-16.1438, -10.5298)
  line L620 (-16.1438, -10.5298) -> (-16.0287, -10.4125)
  line L621 (-16.0287, -10.4125) -> (-15.9954, -10.3717)
  line L622 (-15.9954, -10.3717) -> (-15.9707, -10.3342)
  line L623 (-15.9707, -10.3342) -> (-15.9544, -10.3004)
  line L624 (-15.9544, -10.3004) -> (-15.9466, -10.2706)
  line L625 (-15.9466, -10.2706) -> (-15.9468, -10.2452)
  line L626 (-15.9468, -10.2452) -> (-15.9551, -10.2244)
  line L627 (-15.9551, -10.2244) -> (-15.9733, -10.196)
  line L628 (-15.9733, -10.196) -> (-16.1575, -9.9014)
  line L629 (-16.1575, -9.9014) -> (-16.3364, -9.6034)
  line L630 (-16.3364, -9.6034) -> (-16.3534, -9.5743)
  line L631 (-16.3534, -9.5743) -> (-16.3682, -9.5575)
  line L632 (-16.3682, -9.5575) -> (-16.3908, -9.5457)
  line L633 (-16.3908, -9.5457) -> (-16.4209, -9.5392)
  line L634 (-16.4209, -9.5392) -> (-16.4584, -9.5383)
  line L635 (-16.4584, -9.5383) -> (-16.503, -9.5433)
  line L636 (-16.503, -9.5433) -> (-16.5545, -9.5545)
  line L637 (-16.5545, -9.5545) -> (-16.7112, -9.6038)
  line L638 (-16.7112, -9.6038) -> (-16.9003, -9.6574)
  line L639 (-16.9003, -9.6574) -> (-17.1235, -9.7107)
  line L640 (-17.1235, -9.7107) -> (-17.3806, -9.7608)
  line L641 (-17.3806, -9.7608) -> (-17.6718, -9.805)
  line L642 (-17.6718, -9.805) -> (-17.8299, -9.8239)
  line L643 (-17.8299, -9.8239) -> (-17.9976, -9.8405)
  line L644 (-17.9976, -9.8405) -> (-18.1718, -9.8541)
  line L645 (-18.1718, -9.8541) -> (-18.3579, -9.8647)
  line L646 (-18.3579, -9.8647) -> (-18.5354, -9.8711)
  arc A19 (-18.8807, -9.1934) -> (-18.5354, -9.8711) centre (0, 0) ccw
  line L647 (-18.8807, -9.1934) -> (-18.7712, -9.0535)
  line L648 (-18.7712, -9.0535) -> (-18.6532, -8.9092)
  line L649 (-18.6532, -8.9092) -> (-18.5399, -8.7763)
  line L650 (-18.5399, -8.7763) -> (-18.4279, -8.6503)
  line L651 (-18.4279, -8.6503) -> (-18.3196, -8.5336)
  line L652 (-18.3196, -8.5336) -> (-18.1127, -8.324)
  line L653 (-18.1127, -8.324) -> (-17.9211, -8.1454)
  line L654 (-17.9211, -8.1454) -> (-17.7468, -7.9961)
  line L655 (-17.7468, -7.9961) -> (-17.5923, -7.8747)
  line L656 (-17.5923, -7.8747) -> (-17.4603, -7.7769)
  line L657 (-17.4603, -7.7769) -> (-17.4209, -7.7418)
  line L658 (-17.4209, -7.7418) -> (-17.3907, -7.7086)
  line L659 (-17.3907, -7.7086) -> (-17.3694, -7.6778)
  line L660 (-17.3694, -7.6778) -> (-17.3569, -7.6496)
  line L661 (-17.3569, -7.6496) -> (-17.3532, -7.6244)
  line L662 (-17.3532, -7.6244) -> (-17.3581, -7.6026)
  line L663 (-17.3581, -7.6026) -> (-17.3717, -7.5717)
  line L664 (-17.3717, -7.5717) -> (-17.5075, -7.2519)
  line L665 (-17.5075, -7.2519) -> (-17.6376, -6.9296)
  line L666 (-17.6376, -6.9296) -> (-17.6499, -6.8982)
  line L667 (-17.6499, -6.8982) -> (-17.6618, -6.8793)
  line L668 (-17.6618, -6.8793) -> (-17.6823, -6.8641)
  line L669 (-17.6823, -6.8641) -> (-17.711, -6.853)
  line L670 (-17.711, -6.853) -> (-17.7479, -6.8462)
  line L671 (-17.7479, -6.8462) -> (-17.7927, -6.8442)
  line L672 (-17.7927, -6.8442) -> (-17.8453, -6.8472)
  line L673 (-17.8453, -6.8472) -> (-18.0079, -6.8714)
  line L674 (-18.0079, -6.8714) -> (-18.203, -6.8948)
  line L675 (-18.203, -6.8948) -> (-18.4318, -6.9124)
  line L676 (-18.4318, -6.9124) -> (-18.6935, -6.9217)
  line L677 (-18.6935, -6.9217) -> (-18.9881, -6.9198)
  line L678 (-18.9881, -6.9198) -> (-19.1471, -6.9138)
  line L679 (-19.1471, -6.9138) -> (-19.3155, -6.9039)
  line L680 (-19.3155, -6.9039) -> (-19.4896, -6.8901)
  line L681 (-19.4896, -6.8901) -> (-19.675, -6.8714)
  line L682 (-19.675, -6.8714) -> (-19.8514, -6.85)
  arc A20 (-20.0864, -6.1266) -> (-19.8514, -6.85) centre (0, 0) ccw
  line L683 (-20.0864, -6.1266) -> (-19.9563, -6.0056)
  line L684 (-19.9563, -6.0056) -> (-19.8173, -5.8815)
  line L685 (-19.8173, -5.8815) -> (-19.6846, -5.768)
  line L686 (-19.6846, -5.768) -> (-19.5542, -5.661)
  line L687 (-19.5542, -5.661) -> (-19.429, -5.5627)
  line L688 (-19.429, -5.5627) -> (-19.1918, -5.388)
  line L689 (-19.1918, -5.388) -> (-18.9746, -5.2416)
  line L690 (-18.9746, -5.2416) -> (-18.7791, -5.1215)
  line L691 (-18.7791, -5.1215) -> (-18.6076, -5.0257)
  line L692 (-18.6076, -5.0257) -> (-18.4619, -4.9497)
  line L693 (-18.4619, -4.9497) -> (-18.4175, -4.9212)
  line L694 (-18.4175, -4.9212) -> (-18.3824, -4.8932)
  line L695 (-18.3824, -4.8932) -> (-18.3566, -4.8661)
  line L696 (-18.3566, -4.8661) -> (-18.3399, -4.8402)
  line L697 (-18.3399, -4.8402) -> (-18.3323, -4.8159)
  line L698 (-18.3323, -4.8159) -> (-18.3337, -4.7936)
  line L699 (-18.3337, -4.7936) -> (-18.3423, -4.761)
  line L700 (-18.3423, -4.761) -> (-18.4264, -4.4238)
  line L701 (-18.4264, -4.4238) -> (-18.5045, -4.0852)
  line L702 (-18.5045, -4.0852) -> (-18.5117, -4.0522)
  line L703 (-18.5117, -4.0522) -> (-18.5205, -4.0317)
  line L704 (-18.5205, -4.0317) -> (-18.5383, -4.0135)
  line L705 (-18.5383, -4.0135) -> (-18.565, -3.998)
  line L706 (-18.565, -3.998) -> (-18.6003, -3.9856)
  line L707 (-18.6003, -3.9856) -> (-18.6443, -3.9765)
  line L708 (-18.6443, -3.9765) -> (-18.6968, -3.9713)
  line L709 (-18.6968, -3.9713) -> (-18.8611, -3.9697)
  line L710 (-18.8611, -3.9697) -> (-19.0574, -3.9623)
  line L711 (-19.0574, -3.9623) -> (-19.2862, -3.944)
  line L712 (-19.2862, -3.944) -> (-19.5462, -3.9122)
  line L713 (-19.5462, -3.9122) -> (-19.8368, -3.8642)
  line L714 (-19.8368, -3.8642) -> (-19.993, -3.8334)
  line L715 (-19.993, -3.8334) -> (-20.1577, -3.7973)
  line L716 (-20.1577, -3.7973) -> (-20.3275, -3.7564)
  line L717 (-20.3275, -3.7564) -> (-20.5077, -3.709)
  line L718 (-20.5077, -3.709) -> (-20.6786, -3.6602)
  arc A21 (-20.7975, -2.909) -> (-20.6786, -3.6602) centre (0, 0) ccw
  line L719 (-20.7975, -2.909) -> (-20.6501, -2.8098)
  line L720 (-20.6501, -2.8098) -> (-20.4934, -2.709)
  line L721 (-20.4934, -2.709) -> (-20.3445, -2.6176)
  line L722 (-20.3445, -2.6176) -> (-20.199, -2.5324)
  line L723 (-20.199, -2.5324) -> (-20.06, -2.4549)
  line L724 (-20.06, -2.4549) -> (-19.7984, -2.3194)
  line L725 (-19.7984, -2.3194) -> (-19.561, -2.2088)
  line L726 (-19.561, -2.2088) -> (-19.3491, -2.1207)
  line L727 (-19.3491, -2.1207) -> (-19.1647, -2.053)
  line L728 (-19.1647, -2.053) -> (-19.0089, -2.0007)
  line L729 (-19.0089, -2.0007) -> (-18.9606, -1.9795)
  line L730 (-18.9606, -1.9795) -> (-18.9216, -1.9573)
  line L731 (-18.9216, -1.9573) -> (-18.8918, -1.9346)
  line L732 (-18.8918, -1.9346) -> (-18.8713, -1.9116)
  line L733 (-18.8713, -1.9116) -> (-18.8599, -1.8888)
  line L734 (-18.8599, -1.8888) -> (-18.8579, -1.8665)
  line L735 (-18.8579, -1.8665) -> (-18.8612, -1.833)
  line L736 (-18.8612, -1.833) -> (-18.8916, -1.4868)
  line L737 (-18.8916, -1.4868) -> (-18.9157, -1.1401)
  line L738 (-18.9157, -1.1401) -> (-18.9177, -1.1065)
  line L739 (-18.9177, -1.1065) -> (-18.9232, -1.0848)
  line L740 (-18.9232, -1.0848) -> (-18.938, -1.0641)
  line L741 (-18.938, -1.0641) -> (-18.9618, -1.0446)
  line L742 (-18.9618, -1.0446) -> (-18.9948, -1.0268)
  line L743 (-18.9948, -1.0268) -> (-19.0368, -1.011)
  line L744 (-19.0368, -1.011) -> (-19.0878, -0.9976)
  line L745 (-19.0878, -0.9976) -> (-19.2499, -0.9703)
  line L746 (-19.2499, -0.9703) -> (-19.4426, -0.9323)
  line L747 (-19.4426, -0.9323) -> (-19.6657, -0.8784)
  line L748 (-19.6657, -0.8784) -> (-19.9175, -0.8063)
  line L749 (-19.9175, -0.8063) -> (-20.1971, -0.7135)
  line L750 (-20.1971, -0.7135) -> (-20.3465, -0.6586)
  line L751 (-20.3465, -0.6586) -> (-20.5035, -0.5972)
  line L752 (-20.5035, -0.5972) -> (-20.6649, -0.5302)
  line L753 (-20.6649, -0.5302) -> (-20.8354, -0.4552)
  line L754 (-20.8354, -0.4552) -> (-20.9966, -0.3803)
  arc A22 (-20.9966, 0.3803) -> (-20.9966, -0.3803) centre (0, 0) ccw
  line L755 (-20.9966, 0.3803) -> (-20.8354, 0.4552)
  line L756 (-20.8354, 0.4552) -> (-20.6649, 0.5302)
  line L757 (-20.6649, 0.5302) -> (-20.5035, 0.5972)
  line L758 (-20.5035, 0.5972) -> (-20.3465, 0.6586)
  line L759 (-20.3465, 0.6586) -> (-20.1971, 0.7134)
  line L760 (-20.1971, 0.7134) -> (-19.9175, 0.8063)
  line L761 (-19.9175, 0.8063) -> (-19.6657, 0.8784)
  line L762 (-19.6657, 0.8784) -> (-19.4426, 0.9323)
  line L763 (-19.4426, 0.9323) -> (-19.2499, 0.9703)
  line L764 (-19.2499, 0.9703) -> (-19.0878, 0.9976)
  line L765 (-19.0878, 0.9976) -> (-19.0368, 1.011)
  line L766 (-19.0368, 1.011) -> (-18.9948, 1.0268)
  line L767 (-18.9948, 1.0268) -> (-18.9618, 1.0446)
  line L768 (-18.9618, 1.0446) -> (-18.938, 1.0641)
  line L769 (-18.938, 1.0641) -> (-18.9232, 1.0848)
  line L770 (-18.9232, 1.0848) -> (-18.9177, 1.1065)
  line L771 (-18.9177, 1.1065) -> (-18.9157, 1.1401)
  line L772 (-18.9157, 1.1401) -> (-18.8916, 1.4868)
  line L773 (-18.8916, 1.4868) -> (-18.8612, 1.833)
  line L774 (-18.8612, 1.833) -> (-18.8579, 1.8665)
  line L775 (-18.8579, 1.8665) -> (-18.8599, 1.8888)
  line L776 (-18.8599, 1.8888) -> (-18.8713, 1.9116)
  line L777 (-18.8713, 1.9116) -> (-18.8918, 1.9346)
  line L778 (-18.8918, 1.9346) -> (-18.9216, 1.9573)
  line L779 (-18.9216, 1.9573) -> (-18.9606, 1.9795)
  line L780 (-18.9606, 1.9795) -> (-19.0089, 2.0007)
  line L781 (-19.0089, 2.0007) -> (-19.1647, 2.0529)
  line L782 (-19.1647, 2.0529) -> (-19.3491, 2.1207)
  line L783 (-19.3491, 2.1207) -> (-19.561, 2.2088)
  line L784 (-19.561, 2.2088) -> (-19.7984, 2.3194)
  line L785 (-19.7984, 2.3194) -> (-20.06, 2.4548)
  line L786 (-20.06, 2.4548) -> (-20.199, 2.5324)
  line L787 (-20.199, 2.5324) -> (-20.3445, 2.6176)
  line L788 (-20.3445, 2.6176) -> (-20.4934, 2.709)
  line L789 (-20.4934, 2.709) -> (-20.6501, 2.8098)
  line L790 (-20.6501, 2.8098) -> (-20.7975, 2.909)
  arc A23 (-20.6786, 3.6602) -> (-20.7975, 2.909) centre (0, 0) ccw
  line L791 (-20.6786, 3.6602) -> (-20.5077, 3.7089)
  line L792 (-20.5077, 3.7089) -> (-20.3275, 3.7564)
  line L793 (-20.3275, 3.7564) -> (-20.1577, 3.7973)
  line L794 (-20.1577, 3.7973) -> (-19.993, 3.8334)
  line L795 (-19.993, 3.8334) -> (-19.8368, 3.8642)
  line L796 (-19.8368, 3.8642) -> (-19.5462, 3.9121)
  line L797 (-19.5462, 3.9121) -> (-19.2862, 3.944)
  line L798 (-19.2862, 3.944) -> (-19.0574, 3.9623)
  line L799 (-19.0574, 3.9623) -> (-18.8611, 3.9697)
  line L800 (-18.8611, 3.9697) -> (-18.6968, 3.9713)
  line L801 (-18.6968, 3.9713) -> (-18.6443, 3.9765)
  line L802 (-18.6443, 3.9765) -> (-18.6003, 3.9856)
  line L803 (-18.6003, 3.9856) -> (-18.565, 3.998)
  line L804 (-18.565, 3.998) -> (-18.5383, 4.0135)
  line L805 (-18.5383, 4.0135) -> (-18.5205, 4.0317)
  line L806 (-18.5205, 4.0317) -> (-18.5117, 4.0522)
  line L807 (-18.5117, 4.0522) -> (-18.5045, 4.0851)
  line L808 (-18.5045, 4.0851) -> (-18.4264, 4.4238)
  line L809 (-18.4264, 4.4238) -> (-18.3423, 4.761)
  line L810 (-18.3423, 4.761) -> (-18.3337, 4.7936)
  line L811 (-18.3337, 4.7936) -> (-18.3323, 4.8159)
  line L812 (-18.3323, 4.8159) -> (-18.3399, 4.8402)
  line L813 (-18.3399, 4.8402) -> (-18.3566, 4.8661)
  line L814 (-18.3566, 4.8661) -> (-18.3824, 4.8932)
  line L815 (-18.3824, 4.8932) -> (-18.4175, 4.9212)
  line L816 (-18.4175, 4.9212) -> (-18.4619, 4.9497)
  line L817 (-18.4619, 4.9497) -> (-18.6076, 5.0257)
  line L818 (-18.6076, 5.0257) -> (-18.7791, 5.1215)
  line L819 (-18.7791, 5.1215) -> (-18.9746, 5.2416)
  line L820 (-18.9746, 5.2416) -> (-19.1918, 5.388)
  line L821 (-19.1918, 5.388) -> (-19.429, 5.5627)
  line L822 (-19.429, 5.5627) -> (-19.5542, 5.661)
  line L823 (-19.5542, 5.661) -> (-19.6846, 5.7679)
  line L824 (-19.6846, 5.7679) -> (-19.8173, 5.8815)
  line L825 (-19.8173, 5.8815) -> (-19.9563, 6.0056)
  line L826 (-19.9563, 6.0056) -> (-20.0864, 6.1266)
  arc A24 (-19.8514, 6.85) -> (-20.0864, 6.1266) centre (0, 0) ccw
  line L827 (-19.8514, 6.85) -> (-19.675, 6.8714)
  line L828 (-19.675, 6.8714) -> (-19.4896, 6.8901)
  line L829 (-19.4896, 6.8901) -> (-19.3155, 6.9039)
  line L830 (-19.3155, 6.9039) -> (-19.1471, 6.9138)
  line L831 (-19.1471, 6.9138) -> (-18.9881, 6.9198)
  line L832 (-18.9881, 6.9198) -> (-18.6935, 6.9217)
  line L833 (-18.6935, 6.9217) -> (-18.4318, 6.9124)
  line L834 (-18.4318, 6.9124) -> (-18.203, 6.8947)
  line L835 (-18.203, 6.8947) -> (-18.0079, 6.8714)
  line L836 (-18.0079, 6.8714) -> (-17.8453, 6.8472)
  line L837 (-17.8453, 6.8472) -> (-17.7927, 6.8442)
  line L838 (-17.7927, 6.8442) -> (-17.7479, 6.8462)
  line L839 (-17.7479, 6.8462) -> (-17.711, 6.853)
  line L840 (-17.711, 6.853) -> (-17.6823, 6.8641)
  line L841 (-17.6823, 6.8641) -> (-17.6618, 6.8793)
  line L842 (-17.6618, 6.8793) -> (-17.6499, 6.8982)
  line L843 (-17.6499, 6.8982) -> (-17.6376, 6.9296)
  line L844 (-17.6376, 6.9296) -> (-17.5075, 7.2518)
  line L845 (-17.5075, 7.2518) -> (-17.3716, 7.5717)
  line L846 (-17.3716, 7.5717) -> (-17.3581, 7.6026)
  line L847 (-17.3581, 7.6026) -> (-17.3532, 7.6244)
  line L848 (-17.3532, 7.6244) -> (-17.3569, 7.6496)
  line L849 (-17.3569, 7.6496) -> (-17.3694, 7.6778)
  line L850 (-17.3694, 7.6778) -> (-17.3907, 7.7086)
  line L851 (-17.3907, 7.7086) -> (-17.4209, 7.7418)
  line L852 (-17.4209, 7.7418) -> (-17.4603, 7.7769)
  line L853 (-17.4603, 7.7769) -> (-17.5923, 7.8747)
  line L854 (-17.5923, 7.8747) -> (-17.7468, 7.9961)
  line L855 (-17.7468, 7.9961) -> (-17.9211, 8.1454)
  line L856 (-17.9211, 8.1454) -> (-18.1127, 8.3239)
  line L857 (-18.1127, 8.3239) -> (-18.3196, 8.5336)
  line L858 (-18.3196, 8.5336) -> (-18.4279, 8.6503)
  line L859 (-18.4279, 8.6503) -> (-18.5399, 8.7763)
  line L860 (-18.5399, 8.7763) -> (-18.6532, 8.9092)
  line L861 (-18.6532, 8.9092) -> (-18.7712, 9.0535)
  line L862 (-18.7712, 9.0535) -> (-18.8807, 9.1934)
  arc A25 (-18.5354, 9.8711) -> (-18.8807, 9.1934) centre (0, 0) ccw
  line L863 (-18.5354, 9.8711) -> (-18.3579, 9.8646)
  line L864 (-18.3579, 9.8646) -> (-18.1718, 9.8541)
  line L865 (-18.1718, 9.8541) -> (-17.9976, 9.8405)
  line L866 (-17.9976, 9.8405) -> (-17.8299, 9.8239)
  line L867 (-17.8299, 9.8239) -> (-17.6718, 9.805)
  line L868 (-17.6718, 9.805) -> (-17.3806, 9.7608)
  line L869 (-17.3806, 9.7608) -> (-17.1235, 9.7107)
  line L870 (-17.1235, 9.7107) -> (-16.9003, 9.6574)
  line L871 (-16.9003, 9.6574) -> (-16.7112, 9.6038)
  line L872 (-16.7112, 9.6038) -> (-16.5545, 9.5545)
  line L873 (-16.5545, 9.5545) -> (-16.503, 9.5433)
  line L874 (-16.503, 9.5433) -> (-16.4584, 9.5383)
  line L875 (-16.4584, 9.5383) -> (-16.4209, 9.5392)
  line L876 (-16.4209, 9.5392) -> (-16.3908, 9.5457)
  line L877 (-16.3908, 9.5457) -> (-16.3682, 9.5575)
  line L878 (-16.3682, 9.5575) -> (-16.3534, 9.5743)
  line L879 (-16.3534, 9.5743) -> (-16.3364, 9.6034)
  line L880 (-16.3364, 9.6034) -> (-16.1575, 9.9013)
  line L881 (-16.1575, 9.9013) -> (-15.9733, 10.196)
  line L882 (-15.9733, 10.196) -> (-15.9551, 10.2244)
  line L883 (-15.9551, 10.2244) -> (-15.9468, 10.2452)
  line L884 (-15.9468, 10.2452) -> (-15.9466, 10.2706)
  line L885 (-15.9466, 10.2706) -> (-15.9544, 10.3004)